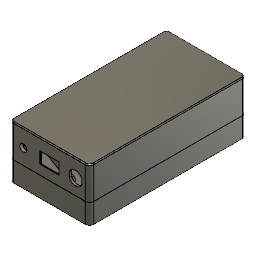
beltpack_pi_2s (Autodesk Fusion 360 design; units mm, degrees)
Autodesk Fusion 360 part; units mm, degrees
note: some values were not read from the file. Set by a fixed rule: which face or edge a step refers to.
sketch "case_form" plane through (0, 0, 0) normal (0, 0, 1) x (1, 0, 0)
  line L0 (0, 0) -> (87, 0)
  line L1 (87, 0) -> (87, 35)
  line L2 (87, 35) -> (0, 35)
  line L3 (0, 35) -> (0, 0)
  dimension "d5" = 87
  dimension "d6" = 35
  measures "d5" distance of L0.start
  measures "d6" distance of L0.start
extrude "Extrude1" add sketch "case_form" along normal blind 175 makes body 1
fillet "Fillet5" radius 2.5 4 edges at (87, 17.5, 175) (0, 17.5, 175) (87, 17.5, 0) (0, 17.5, 0) on bodies 1
shell "Shell1" thickness 2.4 outward yes removed faces 0 bodies 1
fillet "Fillet1" radius 1 8 edges at (-2.4, 37.4, 87.5) (-0.9648, 37.4, -0.9648) (43.5, 37.4, -2.4) (87.9648, 37.4, -0.9648) (89.4, 37.4, 87.5) (87.9648, 37.4, 175.9648) (43.5, 37.4, 177.4) (-0.9648, 37.4, 175.9648) on bodies 1
ref_plane "WorkPlane1" through (43.5, 0, 87.5) normal (0, -1, 0) x (1, 0, 0)
split "Split1" by plane through (43.5, 0, 87.5) normal (0, -1, 0) bodies 1 makes body 2 at (28.2, -2.4, 59.1667)
sketch "electronics" plane through (0, 35, 0) normal (0, -1, 0) x (1, 0, 0)
  line L0 (23, 152) -> (79, 152) construction
  line L1 (79, 152) -> (79, 67) construction
  line L2 (79, 67) -> (23, 67) construction
  line L3 (23, 67) -> (23, 152) construction
  circle A0 centre (26.5, 148.5) radius 3
  circle A1 centre (26.5, 148.5) radius 1
  circle A2 centre (75.5, 148.5) radius 3
  circle A3 centre (75.5, 148.5) radius 1
  circle A4 centre (26.5, 90.5) radius 3
  circle A5 centre (75.5, 90.5) radius 3
  circle A6 centre (75.5, 90.5) radius 1
  circle A7 centre (26.5, 90.5) radius 1
  line L4 (23, 40) -> (50, 40) construction
  line L5 (50, 40) -> (50, 24) construction
  line L6 (50, 24) -> (23, 24) construction
  line L7 (23, 24) -> (23, 40) construction
  circle A8 centre (25, 26) radius 3
  circle A9 centre (25, 26) radius 1
  circle A10 centre (48, 26) radius 3
  circle A11 centre (48, 26) radius 1
  arc A12 (0, 2.5) -> (2.5, 0) centre (2.5, 2.5) ccw
  line L8 (2.5, 0) -> (84.5, 0)
  arc A13 (84.5, 0) -> (87, 2.5) centre (84.5, 2.5) ccw
  line L9 (87, 2.5) -> (87, 172.5)
  arc A14 (87, 172.5) -> (84.5, 175) centre (84.5, 172.5) ccw
  line L10 (84.5, 175) -> (2.5, 175)
  arc A15 (2.5, 175) -> (0, 172.5) centre (2.5, 172.5) ccw
  line L11 (0, 172.5) -> (0, 2.5)
  arc A16 (1.5, 2.5) -> (2.5, 1.5) centre (2.5, 2.5) ccw
  line L12 (2.5, 1.5) -> (84.5, 1.5)
  arc A17 (84.5, 1.5) -> (85.5, 2.5) centre (84.5, 2.5) ccw
  line L13 (85.5, 2.5) -> (85.5, 172.5)
  arc A18 (85.5, 172.5) -> (84.5, 173.5) centre (84.5, 172.5) ccw
  line L14 (84.5, 173.5) -> (2.5, 173.5)
  arc A19 (2.5, 173.5) -> (1.5, 172.5) centre (2.5, 172.5) ccw
  line L15 (1.5, 172.5) -> (1.5, 2.5)
  line L16 (0, 172.5) -> (1.5, 172.5)
  line L17 (1.5, 172.5) -> (1.5, 170.5)
  line L18 (1.5, 170.5) -> (0, 170.5)
  line L19 (0, 170.5) -> (0, 172.5)
  line L20 (2.5, 175) -> (4.5, 175)
  line L21 (4.5, 175) -> (4.5, 173.5)
  line L22 (4.5, 173.5) -> (2.5, 173.5)
  line L23 (2.5, 173.5) -> (2.5, 175)
  arc A20 (0.4999, 2.5) -> (2.5, 0.4999) centre (2.5, 2.5) ccw
  line L24 (2.5, 0.4999) -> (84.5, 0.4999)
  arc A21 (84.5, 0.4999) -> (86.5001, 2.5) centre (84.5, 2.5) ccw
  line L25 (86.5001, 2.5) -> (86.5001, 172.5)
  arc A22 (86.5001, 172.5) -> (84.5, 174.5001) centre (84.5, 172.5) ccw
  line L26 (84.5, 174.5001) -> (2.5, 174.5001)
  arc A23 (2.5, 174.5001) -> (0.4999, 172.5) centre (2.5, 172.5) ccw
  line L27 (0.4999, 172.5) -> (0.4999, 2.5)
  line L28 (84.5, 175) -> (82.5, 175)
  line L29 (82.5, 175) -> (82.5, 138.5)
  line L30 (82.5, 138.5) -> (84.5, 138.5)
  line L31 (84.5, 138.5) -> (84.5, 175)
  line L32 (87, 172.5) -> (85.5, 172.5)
  line L33 (85.5, 172.5) -> (85.5, 170.5)
  line L34 (85.5, 170.5) -> (87, 170.5)
  line L35 (87, 170.5) -> (87, 172.5)
  line L36 (84.5, 0) -> (82.5, 0)
  line L37 (82.5, 0) -> (82.5, 1.5)
  line L38 (82.5, 1.5) -> (84.5, 1.5)
  line L39 (84.5, 1.5) -> (84.5, 0)
  line L40 (87, 2.5) -> (85.5, 2.5)
  line L41 (85.5, 2.5) -> (85.5, 4.5)
  line L42 (85.5, 4.5) -> (87, 4.5)
  line L43 (87, 4.5) -> (87, 2.5)
  line L44 (2.5, 0) -> (4.5, 0)
  line L45 (4.5, 0) -> (4.5, 1.5)
  line L46 (4.5, 1.5) -> (2.5, 1.5)
  line L47 (2.5, 1.5) -> (2.5, 0)
  line L48 (0, 2.5) -> (1.5, 2.5)
  line L49 (1.5, 2.5) -> (1.5, 4.5)
  line L50 (1.5, 4.5) -> (0, 4.5)
  line L51 (0, 4.5) -> (0, 2.5)
  line L52 (85.5, 135) -> (87, 135)
  line L53 (87, 135) -> (87, 130)
  line L54 (87, 130) -> (85.5, 130)
  line L55 (85.5, 130) -> (85.5, 135)
  line L56 (85.5, 45) -> (87, 45)
  line L57 (87, 45) -> (87, 40)
  line L58 (87, 40) -> (85.5, 40)
  line L59 (85.5, 40) -> (85.5, 45)
  line L60 (0, 135) -> (1.5, 135)
  line L61 (1.5, 135) -> (1.5, 130)
  line L62 (1.5, 130) -> (0, 130)
  line L63 (0, 130) -> (0, 135)
  line L64 (1.5, 45) -> (0, 45)
  line L65 (0, 45) -> (0, 40)
  line L66 (0, 40) -> (1.5, 40)
  line L67 (1.5, 40) -> (1.5, 45)
  line L68 (23, 63) -> (54, 63) construction
  line L69 (54, 63) -> (54, 44) construction
  line L70 (54, 44) -> (23, 44) construction
  line L71 (23, 44) -> (23, 63) construction
  circle A24 centre (26, 61) radius 1
  circle A25 centre (26, 61) radius 3
  circle A26 centre (51, 46) radius 1
  circle A27 centre (51, 46) radius 3
  dimension "d12" = 85
  dimension "d13" = 56
  dimension "d15" = 6
  dimension "d16" = 3.5
  dimension "d17" = 3.5
  dimension "d18" = 2
  dimension "d19" = 6
  dimension "d20" = 3.5
  dimension "d21" = 3.5
  dimension "d22" = 2
  dimension "d23" = 6
  dimension "d24" = 6
  dimension "d26" = 3.5
  dimension "d28" = 3.5
  dimension "d29" = 2
  dimension "d30" = 2
  dimension "d114" = 27
  dimension "d115" = 16
  dimension "d118" = 6
  dimension "d120" = 2
  dimension "d121" = 2
  dimension "d122" = 6
  dimension "d125" = 2
  dimension "d357" = 1.5
  dimension "d358" = 2
  dimension "d359" = 1.5
  dimension "d360" = 1.5
  dimension "d361" = 2
  dimension "d366" = 0.4999
  dimension "d375" = 2
  dimension "d376" = 2
  dimension "d377" = 2
  dimension "d378" = 1.5
  dimension "d379" = 1.5
  dimension "d380" = 2
  dimension "d381" = 2
  dimension "d382" = 1.5
  dimension "d383" = 1.5
  dimension "d384" = 2
  dimension "d419" = 5
  dimension "d420" = 40
  dimension "d422" = 5
  dimension "d423" = 85
  dimension "d425" = 1.5
  dimension "d426" = 5
  dimension "d427" = 40
  dimension "d428" = 5
  dimension "d429" = 1.5
  dimension "d430" = 85
  dimension "d490" = 58
  dimension "d491" = 58
  dimension "d492" = 26.5
  dimension "d493" = 26.5
  dimension "d494" = 22
  dimension "d495" = 19
  dimension "d496" = 31
  dimension "d497" = 2
  dimension "d498" = 6
  dimension "d499" = 2
  dimension "d500" = 2
  dimension "d501" = 6
  dimension "d502" = 2
  dimension "d503" = 3
  dimension "d504" = 3
  dimension "d505" = 4
  dimension "d507" = 2
  dimension "d508" = 4
  dimension "d509" = 2
  dimension "d510" = 2
  measures "d15" diameter of A0
  measures "d18" diameter of A1
  measures "d19" diameter of A2
  measures "d22" diameter of A3
  measures "d23" diameter of A4
  measures "d24" diameter of A5
  measures "d29" diameter of A6
  measures "d30" diameter of A7
  measures "d118" diameter of A8
  measures "d121" diameter of A9
  measures "d122" diameter of A10
  measures "d125" diameter of A11
  measures "d359" distance of origin
  measures "d378" distance of origin
  measures "d425" distance of origin
  measures "d427" distance of L10
  measures "d492" distance of origin L10
  measures "d493" distance of origin L11
  measures "d497" diameter of A24
  measures "d498" diameter of A25
  measures "d500" diameter of A26
  measures "d501" diameter of A27
  measures "d505" distance of L2 L68
  measures "d508" distance of L4 L70
sketch "oled_panel" plane through (0, 0, 177.4) normal (0, 0, 1) x (1, 0, 0)
  line L0 (2.5, 0) -> (84.5, 0)
  line L1 (29.5, 33.7) -> (57.5, 33.7)
  line L2 (57.5, 33.7) -> (57.5, 5.2)
  line L3 (57.5, 5.2) -> (29.5, 5.2)
  line L4 (29.5, 5.2) -> (29.5, 33.7)
  line L5 (32.5, 24) -> (54.5, 24)
  line L6 (54.5, 24) -> (54.5, 11)
  line L7 (54.5, 11) -> (32.5, 11)
  line L8 (32.5, 11) -> (32.5, 24)
  line L9 (43.5, 24) -> (43.5, 11) construction
  line L10 (54.5, 17.5) -> (32.5, 17.5) construction
  circle A0 centre (13.6, 17.5) radius 4
  circle A1 centre (73.4, 17.5) radius 7.75
  line L11 (28.5, 34.7) -> (20.7, 34.7)
  line L12 (20.7, 34.7) -> (20.7, 26.9)
  line L13 (20.7, 26.9) -> (28.5, 26.9)
  line L14 (28.5, 26.9) -> (28.5, 34.7)
  line L15 (24.6, 34.7) -> (24.6, 19.5918)
  line L16 (24.6, 19.5918) -> (24.6, 26.9) construction
  line L17 (20.7, 30.8) -> (28.5, 30.8) construction
  line L18 (58.5, 12) -> (66.3, 12)
  line L19 (66.3, 12) -> (66.3, 4.2)
  line L20 (66.3, 4.2) -> (58.5, 4.2)
  line L21 (58.5, 4.2) -> (58.5, 12)
  line L22 (62.4, 12) -> (62.4, 4.2) construction
  line L23 (66.3, 8.1) -> (58.5, 8.1) construction
  circle A2 centre (24.6, 30.8) radius 1.6
  circle A3 centre (24.6, 30.8) radius 1
  circle A4 centre (62.4, 8.1) radius 1.6
  circle A5 centre (62.4, 8.1) radius 1
  line L24 (66.25, 23.5) -> (80.55, 23.5)
  line L25 (80.55, 23.5) -> (80.55, 11.5)
  line L26 (80.55, 11.5) -> (66.25, 11.5)
  line L27 (66.25, 11.5) -> (66.25, 23.5)
  line L28 (66.25, 17.5) -> (80.55, 17.5) construction
  line L29 (73.4, 23.5) -> (73.4, 11.5) construction
  line L30 (7.3498, 14.0837) -> (9.2554, 11.7666)
  line L31 (9.2554, 11.7666) -> (7.7223, 10.4776)
  line L32 (7.7223, 10.4776) -> (5.8047, 12.8137)
  line L33 (5.8047, 12.8137) -> (7.3498, 14.0837)
  circle A6 centre (13.6, 17.5) radius 8.2 construction
  line L34 (8.3026, 12.9251) -> (6.7635, 11.6457) construction
  line L35 (6.5772, 13.4487) -> (8.4888, 11.1221) construction
  line L36 (30, 8.45) -> (35.5, 8.45)
  line L37 (35.5, 8.45) -> (35.5, 5.7)
  line L38 (35.5, 5.7) -> (30, 5.7)
  line L39 (30, 5.7) -> (30, 8.45)
  line L40 (79, 35) -> (23, 35)
  line L41 (43.5, 0) -> (43.5, 35)
  line L42 (84.5, 0) -> (84.5, 36.4)
  line L43 (84.5, 36.4) -> (2.5, 36.4)
  line L44 (2.5, 36.4) -> (2.5, 0)
  line L45 (58.5, 34.7) -> (58.5, 4.2)
  line L46 (58.5, 4.2) -> (28.5, 4.2)
  line L47 (28.5, 4.2) -> (28.5, 34.7)
  line L48 (28.5, 34.7) -> (58.5, 34.7)
  line L49 (51.5, 8.45) -> (57, 8.45)
  line L50 (57, 8.45) -> (57, 5.7)
  line L51 (57, 5.7) -> (51.5, 5.7)
  line L52 (51.5, 5.7) -> (51.5, 8.45)
  line L53 (38.15, 7.7) -> (48.85, 7.7)
  line L54 (48.85, 7.7) -> (48.85, 5.7)
  line L55 (48.85, 5.7) -> (38.15, 5.7)
  line L56 (38.15, 5.7) -> (38.15, 7.7)
  line L57 (30, 33.2) -> (35.5, 33.2)
  line L58 (35.5, 33.2) -> (35.5, 30.45)
  line L59 (35.5, 30.45) -> (30, 30.45)
  line L60 (30, 30.45) -> (30, 33.2)
  line L61 (51.5, 33.2) -> (57, 33.2)
  line L62 (57, 33.2) -> (57, 30.45)
  line L63 (57, 30.45) -> (51.5, 30.45)
  line L64 (51.5, 30.45) -> (51.5, 33.2)
  line L65 (19.2644, 29.4032) -> (25.9968, 25.4644)
  line L66 (25.9968, 25.4644) -> (29.9356, 32.1968)
  line L67 (29.9356, 32.1968) -> (23.2032, 36.1356)
  line L68 (23.2032, 36.1356) -> (19.2644, 29.4032)
  line L69 (27.9662, 28.8306) -> (21.2338, 32.7694) construction
  line L70 (22.6306, 27.4338) -> (26.5694, 34.1662) construction
  circle A7 centre (24.6, 30.8) radius 1.6
  line L71 (57.0638, 6.736) -> (63.7686, 2.7504)
  line L72 (63.7686, 2.7504) -> (67.7338, 9.4635)
  line L73 (67.7338, 9.4635) -> (61.0338, 13.4501)
  line L74 (61.0338, 13.4501) -> (57.0638, 6.736)
  line L75 (59.0488, 10.0931) -> (65.7512, 6.1069) construction
  line L76 (60.4162, 4.7432) -> (64.3838, 11.4568) construction
  circle A8 centre (62.4, 8.1) radius 1.6
  line L77 (25.9968, 25.4644) -> (57.0918, 6.7188)
  line L78 (57.0918, 6.7188) -> (61.0338, 13.4501)
  line L79 (61.0338, 13.4501) -> (29.936, 32.1974)
  line L80 (29.936, 32.1974) -> (25.9968, 25.4644)
  line L81 (73.4, 0) -> (73.4, 35) construction
  circle A9 centre (73.4, 17.5) radius 10.5 construction
  line L82 (62.4, 12) -> (66.3, 8.1)
  circle A10 centre (13.6, 17.5) radius 10
  dimension "d31" = 28
  dimension "d32" = 28.5
  dimension "d33" = 22
  dimension "d34" = 13
  dimension "d36" = 8
  dimension "d38" = 1
  dimension "d39" = 15.5
  dimension "d40" = 7.8
  dimension "d41" = 7.8
  dimension "d42" = 7.8
  dimension "d43" = 7.8
  dimension "d44" = 3.2
  dimension "d45" = 2
  dimension "d46" = 3.2
  dimension "d47" = 2
  dimension "d50" = 5.8
  dimension "d51" = 14.3
  dimension "d52" = 12
  dimension "d53" = 3
  dimension "d54" = 2
  dimension "d55" = 16.4
  dimension "d57" = 5.5
  dimension "d58" = 2.75
  dimension "d59" = 0.5
  dimension "d60" = 0.5
  dimension "d80" = 8
  dimension "d451" = 5.5
  dimension "d452" = 2.75
  dimension "d453" = 0.5
  dimension "d454" = 0.5
  dimension "d455" = 10.7
  dimension "d456" = 2
  dimension "d457" = 0.5
  dimension "d458" = 5.5
  dimension "d459" = 2.75
  dimension "d460" = 0.5
  dimension "d461" = 0.5
  dimension "d462" = 5.5
  dimension "d463" = 2.75
  dimension "d464" = 0.5
  dimension "d465" = 0.5
  dimension "d472" = 7.8
  dimension "d473" = 7.8
  dimension "d474" = 3.2
  dimension "d475" = 7.8
  dimension "d476" = 7.8
  dimension "d477" = 3.2
  dimension "d479" = 7.8
  dimension "d487" = 11.1
  dimension "d488" = 21
  dimension "d512" = 20
  measures "d32" distance of origin
  measures "d34" distance of origin
  measures "d36" diameter of A0
  measures "d38" distance of L2
  measures "d39" diameter of A1
  measures "d44" diameter of A2
  measures "d45" diameter of A3
  measures "d46" diameter of A4
  measures "d47" diameter of A5
  measures "d50" distance of L3 L7
  measures "d52" distance of origin
  measures "d55" diameter of A6
  measures "d59" distance of L3 L38
  measures "d60" distance of L4 L39
  measures "d453" distance of L3 L51
  measures "d454" distance of L2 L50
  measures "d457" distance of L3 L55
  measures "d460" distance of L1 L57
  measures "d461" distance of L4 L60
  measures "d464" distance of L1 L61
  measures "d465" distance of L2 L62
  measures "d472" distance of origin
  measures "d473" distance of origin
  measures "d474" diameter of A7
  measures "d477" diameter of A8
  measures "d479" distance of L77 L79
  measures "d488" diameter of A9
  measures "d512" diameter of A10
extrude "Extrude2" cut sketch "oled_panel" against normal up to surface (2.4 mm away) contours L5 L8 L41 L77 | L5 L6 L7 L41 L77 L79 | L5 L6 L79 | L7 L41 L77 | L7 L8 L41 L77 | A1 L24 L25 L26 L27 | A1 L26 | A1 L24 | A0 bodies 1
extrude "Extrude3" cut sketch "electronics" against normal blind 1 contours A1 | A3 | A6 | A7 | A9 | A11 | A24 | A26 bodies 1
extrude "Extrude4" add sketch "electronics" along normal blind 5 contours A0 | A2 | A4 | A5 | A8 | A10 | A25 | A27 bodies 1
extrude "Extrude7" cut sketch "oled_panel" along normal blind 1.4 from surface at -2.4 contours L1 L4 L41 L57 L58 L59 L60 L67 L79 | L1 L2 L5 L6 L41 L79 | L4 L66 L67 L80 | L5 L41 L79 | L4 L5 L8 L41 L59 L60 L66 L77 L79 L80 | L2 L6 L7 L49 L50 L74 L77 L79 | L57 L58 L59 L60 L79 | L59 L60 L79 | L3 L4 L7 L8 L41 L53 L55 L56 L77 | L2 L71 L74 L77 L78 | L2 L71 L78 | L2 L3 L7 L41 L49 L50 L51 L52 L53 L54 L55 L71 L77 | L49 L50 L77 | L49 L50 L51 L52 L77 | L41 L53 L54 L55 | L41 L53 L55 L56 | L36 L37 L38 L39 | L61 L62 L63 L64 bodies 1
extrude "Extrude8" add sketch "oled_panel" against normal blind 2.6 from surface at -2.4 contours L1 L4 L14 L41 L47 L48 L67 | L1 L2 L41 L45 L48 L79 | L4 L14 L47 L66 L67 L80 | L4 L14 L47 L66 L77 L80 | L11 L14 L47 L67 | L11 L13 L14 L15 A2 L47 L66 L67 A7 L80 | L2 L21 L45 L74 L79 | L3 L4 L41 L46 L47 L77 | L13 L14 L47 L66 L80 | L2 L21 L45 L74 L78 | L11 L12 L13 L15 A2 L65 L68 A7 | L2 L21 L45 L71 L78 | L18 L21 L45 L74 L78 | L18 L21 L45 L74 | L2 L3 L21 L41 L45 L46 L71 | L11 L12 L68 | L15 A2 A3 A7 | L15 A2 A3 A7 | L18 L19 L20 L21 L45 L71 L72 L78 L82 | L12 L13 L65 | L20 L21 L45 L71 | L19 L20 L72 | A4 A8 bodies 1
fillet "Fillet3" radius 2 9 edges at (28.5, 4.2, 173.7) (66.3, 4.2, 173.7) (20.7, 26.9, 173.7) (58.5, 12, 173.7) (58.5, 34.7, 173.7) (28.5, 26.9, 173.7) (20.7, 34.7, 173.7) (62.4, 12, 173.7) (66.3, 8.1, 173.7) on bodies 1
extrude "Extrude36" add sketch "oled_panel" against normal blind 2.5 contours L57 L58 L59 L60 L79 | L59 L60 L79 | L49 L50 L77 | L49 L50 L51 L52 L77 | L36 L37 L38 L39 | L61 L62 L63 L64 bodies 1
fillet "Fillet18" radius 1 16 edges at (51.5, 8.45, 175.65) (57, 8.45, 175.65) (51.5, 5.7, 175.65) (57, 5.7, 175.65) (35.5, 8.45, 175.65) (35.5, 5.7, 175.65) (30, 8.45, 175.65) (30, 5.7, 175.65) (30, 30.45, 175.65) (35.5, 30.45, 175.65) (35.5, 33.2, 175.65) (30, 33.2, 175.65) (51.5, 33.2, 175.65) (51.5, 30.45, 175.65) (57, 33.2, 175.65) (57, 30.45, 175.65) on bodies 1
sketch "headset_panel" plane through (0, 0, -2.4) normal (0, 0, -1) x (-1, 0, 0)
  line L0 (-84.5, 0) -> (-2.5, 0)
  line L1 (-39, 31.7) -> (-8, 31.7) construction
  line L2 (-8, 31.7) -> (-8, 5.7) construction
  line L3 (-8, 5.7) -> (-39, 5.7) construction
  line L4 (-39, 5.7) -> (-39, 31.7) construction
  line L5 (-87, 0) -> (-87, 35)
  line L6 (-39, 18.7) -> (-8, 18.7) construction
  line L7 (-23.5, 31.7) -> (-23.5, 5.7) construction
  circle A0 centre (-23.5, 18.7) radius 12.3
  circle A1 centre (-35.6, 8.9) radius 1.6
  circle A2 centre (-11.4, 28.5) radius 1.6
  circle A3 centre (-47, 18.7) radius 4.1
  line L8 (0, 0) -> (0, 35)
  line L9 (-2.5, 0) -> (-2.5, 36.4)
  line L10 (-2.5, 36.4) -> (-84.5, 36.4)
  line L11 (-84.5, 36.4) -> (-84.5, 0)
  line L12 (-30, 0) -> (-24, 0)
  line L13 (-24, 0) -> (-24, 5.2)
  line L14 (-24, 5.2) -> (-30, 5.2)
  line L15 (-30, 5.2) -> (-30, 0)
  line L16 (-8, -2) -> (-79, -2)
  line L17 (-79, -2) -> (-79, 0)
  line L18 (-79, 0) -> (-8, 0)
  line L19 (-8, 0) -> (-8, -2)
  line L20 (-24, 0) -> (-30, 0)
  line L21 (-30, 0) -> (-30, -2)
  line L22 (-30, -2) -> (-24, -2)
  line L23 (-24, -2) -> (-24, 0)
  line L24 (-79, -2) -> (-8, -2)
  line L25 (-8, -2) -> (-8, -7)
  line L26 (-8, -7) -> (-79, -7)
  line L27 (-79, -7) -> (-79, -2)
  line L28 (-10, -7) -> (-77, -7)
  line L29 (-77, -7) -> (-77, -1)
  line L30 (-77, -1) -> (-10, -1)
  line L31 (-10, -1) -> (-10, -7)
  dimension "d82" = 31
  dimension "d83" = 26
  dimension "d89" = 24.6
  dimension "d90" = 3.2
  dimension "d91" = 3.2
  dimension "d92" = 3.4
  dimension "d93" = 3.2
  dimension "d94" = 3.2
  dimension "d95" = 3.4
  dimension "d96" = 8.2
  dimension "d101" = 8
  dimension "d102" = 8
  dimension "d230" = 6
  dimension "d231" = 5.2
  dimension "d302" = 4.7
  dimension "d308" = 24
  dimension "d350" = 71
  dimension "d351" = 2
  dimension "d398" = 5
  dimension "d399" = 67
  dimension "d401" = 6
  dimension "d450" = 6
  measures "d82" distance of L8.start
  measures "d83" distance of L8.start
  measures "d89" diameter of A0
  measures "d90" diameter of A1
  measures "d91" distance of L3
  measures "d92" distance of L4
  measures "d93" diameter of A2
  measures "d94" distance of L1
  measures "d95" distance of L2
  measures "d96" diameter of A3
  measures "d230" distance of L8.start
  measures "d231" distance of L8.start
  measures "d302" distance of L8.start L10
  measures "d308" distance of L8 L13
  measures "d399" distance of L29 L31
  measures "d401" distance of L28 L30
  measures "d450" distance of L21 L23
extrude "Extrude9" cut sketch "headset_panel" against normal up to surface (2.4 mm away) contours L0 L12 L13 L14 L15 L18 L20 | A0 | A1 | A2 | A3 bodies 1
sketch "mounting bosses" plane through (0, -2.4, 0) normal (0, -1, 0) x (1, 0, 0)
  arc A0 (-2.4, 2.5) -> (2.5, -2.4) centre (2.5, 2.5) ccw
  line L0 (2.5, -2.4) -> (84.5, -2.4)
  arc A1 (84.5, -2.4) -> (89.4, 2.5) centre (84.5, 2.5) ccw
  line L1 (89.4, 2.5) -> (89.4, 172.5)
  arc A2 (89.4, 172.5) -> (84.5, 177.4) centre (84.5, 172.5) ccw
  line L2 (84.5, 177.4) -> (2.5, 177.4)
  arc A3 (2.5, 177.4) -> (-2.4, 172.5) centre (2.5, 172.5) ccw
  line L3 (-2.4, 172.5) -> (-2.4, 2.5)
  line L4 (0, 2.5) -> (0, 172.5)
  line L5 (84.5, 0) -> (2.5, 0)
  line L6 (17.6, 175) -> (9.6, 175)
  line L7 (2.5, 175) -> (84.5, 175)
  circle A4 centre (2.6, 160) radius 2.3
  line L8 (0, 165) -> (7.6, 165)
  line L9 (7.6, 165) -> (7.6, 155)
  line L10 (7.6, 155) -> (0, 155)
  line L11 (0, 155) -> (0, 165)
  line L12 (3.8, 155) -> (3.8, 165) construction
  line L13 (0, 20) -> (7.6, 20)
  line L14 (7.6, 20) -> (7.6, 10)
  line L15 (7.6, 10) -> (0, 10)
  line L16 (0, 10) -> (0, 20)
  circle A5 centre (2.6, 15) radius 2.3
  line L17 (3.8, 10) -> (3.8, 20) construction
  circle A6 centre (2.6, 87.5) radius 2.3
  line L18 (0, 92.5) -> (7.6, 92.5)
  line L19 (7.6, 92.5) -> (7.6, 82.5)
  line L20 (7.6, 82.5) -> (0, 82.5)
  line L21 (0, 82.5) -> (0, 92.5)
  line L22 (3.8, 82.5) -> (3.8, 92.5) construction
  circle A7 centre (84.4, 15) radius 2.3
  line L23 (87, 10) -> (79.4, 10)
  line L24 (79.4, 10) -> (79.4, 20)
  line L25 (79.4, 20) -> (87, 20)
  line L26 (87, 20) -> (87, 10)
  line L27 (87, 2.5) -> (87, 172.5)
  line L28 (83.2, 10) -> (83.2, 20) construction
  circle A8 centre (84.4, 87.5) radius 2.3
  line L29 (87, 82.5) -> (79.4, 82.5)
  line L30 (79.4, 82.5) -> (79.4, 92.5)
  line L31 (79.4, 92.5) -> (87, 92.5)
  line L32 (87, 92.5) -> (87, 82.5)
  line L33 (83.2, 82.5) -> (83.2, 92.5) construction
  line L34 (87, 165) -> (79.4, 165)
  line L35 (79.4, 165) -> (79.4, 155)
  line L36 (79.4, 155) -> (87, 155)
  line L37 (87, 155) -> (87, 165)
  circle A9 centre (84.4, 160) radius 2.3
  line L38 (83.2, 155) -> (83.2, 165) construction
  line L39 (30, 0) -> (84.5, 0)
  line L40 (2.5, 0) -> (24, 0)
  line L41 (2.5, 0.6) -> (84.5, 0.6)
  arc A10 (84.5, 0.6) -> (86.4, 2.5) centre (84.5, 2.5) ccw
  line L42 (86.4, 2.5) -> (86.4, 172.5)
  arc A11 (86.4, 172.5) -> (84.5, 174.4) centre (84.5, 172.5) ccw
  line L43 (84.5, 174.4) -> (2.5, 174.4)
  arc A12 (2.5, 174.4) -> (0.6, 172.5) centre (2.5, 172.5) ccw
  line L44 (0.6, 172.5) -> (0.6, 2.5)
  arc A13 (0.6, 2.5) -> (2.5, 0.6) centre (2.5, 2.5) ccw
  dimension "d149" = 4.6
  dimension "d150" = 5
  dimension "d151" = 7.6
  dimension "d152" = 10
  dimension "d153" = 10
  dimension "d160" = 7.6
  dimension "d161" = 10
  dimension "d162" = 4.6
  dimension "d163" = 5
  dimension "d164" = 10
  dimension "d166" = 4.6
  dimension "d167" = 5
  dimension "d168" = 10
  dimension "d169" = 7.6
  dimension "d173" = 4.6
  dimension "d174" = 5
  dimension "d175" = 7.6
  dimension "d176" = 10
  dimension "d178" = 4.6
  dimension "d179" = 5
  dimension "d180" = 10
  dimension "d181" = 7.6
  dimension "d182" = 7.6
  dimension "d183" = 10
  dimension "d184" = 4.6
  dimension "d185" = 5
  dimension "d186" = 10
  dimension "d188" = 3
  measures "d149" diameter of A4
  measures "d150" distance of L3
  measures "d153" distance of L7 L8
  measures "d162" diameter of A5
  measures "d163" distance of L3
  measures "d164" distance of L5
  measures "d166" diameter of A6
  measures "d173" diameter of A7
  measures "d174" distance of L1
  measures "d176" distance of origin
  measures "d178" diameter of A8
  measures "d180" distance of origin
  measures "d181" distance of origin
  measures "d182" distance of origin
  measures "d183" distance of origin
  measures "d184" diameter of A9
  measures "d185" distance of L1 origin
  measures "d186" distance of L7
  measures "d188" distance of L0
extrude "Extrude12" add sketch "mounting bosses" against normal blind 1.6 separate body contours L13 L14 L15 A5 L44 | L8 L9 L10 L13 L14 L15 L18 L19 L20 L23 L24 L25 L29 L30 L31 L34 L35 L36 L41 A10 L42 A11 L43 A12 L44 A13 | A5 L44 | A6 L18 L19 L20 L44 | A6 L44 | A4 L8 L9 L10 L44 | A4 L44 | A7 L23 L24 L25 L42 | A7 L42 | A8 L29 L30 L31 L42 | L34 L35 L36 A9 L42 | A8 L42 | A9 L42 picked at (2.2057, 15.7049) picked at (3.6343, 87.5501) picked at (2.0333, 160) picked at (85.7042, 15.7265) picked at (85.3112, 88.0822) picked at (84.8425, 160) makes body 3
extrude "Extrude11" add sketch "mounting bosses" against normal blind 15 from surface at -4.5 contours L4 L13 L15 L16 A5 L44 | L13 L14 L15 A5 L44 | L4 A6 L18 L20 L21 L44 | A6 L18 L19 L20 L44 | L4 A4 L8 L10 L11 L44 | A4 L8 L9 L10 L44 | A7 L23 L25 L26 L27 L42 | A7 L23 L24 L25 L42 | L27 A8 L29 L31 L32 L42 | A8 L29 L30 L31 L42 | L34 L35 L36 A9 L42 | L27 L34 L36 L37 A9 L42 bodies 1
chamfer "Chamfer2" distance 7.5 angle 45 6 edges at (7.6, 17.1, 160) (7.6, 17.1, 15) (7.6, 17.1, 87.5) (79.4, 17.1, 160) (79.4, 17.1, 87.5) (79.4, 17.1, 15) measured on face at (6.7, 17.1, 160) measured on face at (6.7, 17.1, 15) measured on face at (6.7, 17.1, 87.5) measured on face at (80.3, 17.1, 160) measured on face at (80.3, 17.1, 87.5) measured on face at (80.3, 17.1, 15) on bodies 1
fillet "Fillet6" radius 2 24 edges at (7.6, 5.85, 155) (7.6, 5.85, 165) (0, 9.6, 165) (0, 9.6, 155) (0, 9.6, 20) (7.6, 5.85, 20) (7.6, 5.85, 10) (0, 9.6, 10) (0, 9.6, 82.5) (7.6, 5.85, 82.5) (7.6, 5.85, 92.5) (0, 9.6, 92.5) (87, 9.6, 165) (79.4, 5.85, 165) (79.4, 5.85, 155) (87, 9.6, 92.5) (79.4, 5.85, 92.5) (79.4, 5.85, 82.5) (87, 9.6, 20) (79.4, 5.85, 20) (79.4, 5.85, 10) (87, 9.6, 155) (87, 9.6, 82.5) (87, 9.6, 10) on bodies 1
move_body "Move3" bodies 3 to x (1, 0, 0) y (0, 1, 0) z (0, 0, 1) at (0, 2.8, 0)
sketch "battery_bottom" plane through (0, 0.4, 0) normal (0, -1, 0) x (1, 0, 0)
  arc A0 (0.6, 2.5) -> (2.5, 0.6) centre (2.5, 2.5) ccw
  line L0 (2.5, 0.6) -> (84.5, 0.6)
  arc A1 (84.5, 0.6) -> (86.4, 2.5) centre (84.5, 2.5) ccw
  line L1 (86.4, 2.5) -> (86.4, 172.5)
  arc A2 (86.4, 172.5) -> (84.5, 174.4) centre (84.5, 172.5) ccw
  line L2 (84.5, 174.4) -> (2.5, 174.4)
  arc A3 (2.5, 174.4) -> (0.6, 172.5) centre (2.5, 172.5) ccw
  line L3 (0.6, 172.5) -> (0.6, 2.5)
  line L4 (0.6, 17.6) -> (5.4, 17.6)
  line L5 (5.4, 17.6) -> (5.4, 12.4)
  line L6 (5.4, 12.4) -> (0.6, 12.4)
  line L7 (0.6, 12.4) -> (0.6, 17.6)
  line L8 (3, 12.4) -> (3, 17.6) construction
  line L9 (0.6, 90.1) -> (5.4, 90.1)
  line L10 (5.4, 90.1) -> (5.4, 84.9)
  line L11 (5.4, 84.9) -> (0.6, 84.9)
  line L12 (0.6, 84.9) -> (0.6, 90.1)
  line L13 (3, 90.1) -> (3, 84.9) construction
  line L14 (0.6, 162.6) -> (5.4, 162.6)
  line L15 (5.4, 162.6) -> (5.4, 157.4)
  line L16 (5.4, 157.4) -> (0.6, 157.4)
  line L17 (0.6, 157.4) -> (0.6, 162.6)
  line L18 (3, 157.4) -> (3, 162.6) construction
  line L19 (86.4, 162.6) -> (81.6, 162.6)
  line L20 (81.6, 162.6) -> (81.6, 157.4)
  line L21 (81.6, 157.4) -> (86.4, 157.4)
  line L22 (86.4, 157.4) -> (86.4, 162.6)
  line L23 (84, 162.6) -> (84, 157.4) construction
  line L24 (86.4, 90.1) -> (81.6, 90.1)
  line L25 (81.6, 90.1) -> (81.6, 84.9)
  line L26 (81.6, 84.9) -> (86.4, 84.9)
  line L27 (86.4, 84.9) -> (86.4, 90.1)
  line L28 (84, 84.9) -> (84, 90.1) construction
  line L29 (86.4, 17.6) -> (81.6, 17.6)
  line L30 (81.6, 17.6) -> (81.6, 12.4)
  line L31 (81.6, 12.4) -> (86.4, 12.4)
  line L32 (86.4, 12.4) -> (86.4, 17.6)
  line L33 (84, 12.4) -> (84, 17.6) construction
  line L34 (86.6, 174.4) -> (0.6, 174.4)
  line L35 (0.6, 174.4) -> (0.6, 168.4)
  line L36 (0.6, 168.4) -> (86.6, 168.4)
  line L37 (86.6, 168.4) -> (86.6, 174.4)
  line L38 (30, 0.6) -> (24, 0.6)
  line L39 (24, 0.6) -> (24, 8.1)
  line L40 (24, 8.1) -> (30, 8.1)
  line L41 (30, 8.1) -> (30, 0.6)
  line L42 (0, 2.5) -> (0, 172.5)
  line L43 (0.6, 6) -> (6, 0.6)
  line L44 (81, 0.6) -> (86.4, 6)
  line L45 (0.6, 46.1) -> (2.6, 46.1)
  line L46 (2.6, 46.1) -> (2.6, 39.1)
  line L47 (2.6, 39.1) -> (0.6, 39.1)
  line L48 (0.6, 39.1) -> (0.6, 46.1)
  line L49 (0.6, 136.1) -> (2.6, 136.1)
  line L50 (2.6, 136.1) -> (2.6, 129.1)
  line L51 (2.6, 129.1) -> (0.6, 129.1)
  line L52 (0.6, 129.1) -> (0.6, 136.1)
  line L53 (86.4, 39.1) -> (84.4, 39.1)
  line L54 (84.4, 39.1) -> (84.4, 46.1)
  line L55 (84.4, 46.1) -> (86.4, 46.1)
  line L56 (86.4, 46.1) -> (86.4, 39.1)
  line L57 (86.4, 136.1) -> (84.4, 136.1)
  line L58 (84.4, 136.1) -> (84.4, 129.1)
  line L59 (84.4, 129.1) -> (86.4, 129.1)
  line L60 (86.4, 129.1) -> (86.4, 136.1)
  dimension "d194" = 5.2
  dimension "d195" = 4.8
  dimension "d199" = 5.2
  dimension "d200" = 4.8
  dimension "d201" = 5.2
  dimension "d202" = 4.8
  dimension "d203" = 5.2
  dimension "d204" = 4.8
  dimension "d205" = 4.8
  dimension "d206" = 5.2
  dimension "d207" = 5.2
  dimension "d208" = 4.8
  dimension "d210" = 6
  dimension "d211" = 86
  dimension "d303" = 6
  dimension "d304" = 7.5
  dimension "d309" = 24
  dimension "d391" = 5.4
  dimension "d392" = 5.4
  dimension "d393" = 5.4
  dimension "d394" = 5.4
  dimension "d432" = 7
  dimension "d433" = 2
  dimension "d435" = 38.5
  dimension "d436" = 7
  dimension "d437" = 2
  dimension "d438" = 83
  dimension "d440" = 7
  dimension "d441" = 2
  dimension "d442" = 7
  dimension "d443" = 2
  dimension "d444" = 38.5
  dimension "d445" = 83
  measures "d200" distance of origin
  measures "d202" distance of origin
  measures "d290" distance of origin
  measures "d303" distance of origin
  measures "d304" distance of origin
  measures "d309" distance of L39 L42
  measures "d391" distance of L3
  measures "d392" distance of L0
  measures "d393" distance of L0
  measures "d394" distance of L1 origin
  measures "d433" distance of origin
  measures "d435" distance of L0
  measures "d437" distance of origin
  measures "d444" distance of origin
extrude "Extrude14" cut sketch "battery_bottom" against normal up to surface (1.6 mm away) contours L3 L4 L5 L6 L7 | L3 L9 L10 L11 L12 | L1 L29 L30 L31 L32 | L3 L14 L15 L16 L17 | L1 L24 L25 L26 L27 | L1 L19 L20 L21 L22 bodies 3
extrude "Extrude15" cut sketch "battery_bottom" against normal up to surface (1.6 mm away) contours L1 A2 L2 A3 L3 L34 L35 L36 bodies 3
fillet "Fillet7" radius 2.5 26 edges at (0.6, 1.2, 17.6) (5.4, 1.2, 17.6) (5.4, 1.2, 12.4) (0.6, 1.2, 12.4) (5.4, 1.2, 84.9) (5.4, 1.2, 90.1) (0.6, 1.2, 90.1) (0.6, 1.2, 84.9) (0.6, 1.2, 162.6) (5.4, 1.2, 162.6) (5.4, 1.2, 157.4) (0.6, 1.2, 157.4) (86.4, 1.2, 162.6) (81.6, 1.2, 162.6) (81.6, 1.2, 157.4) (86.4, 1.2, 157.4) (86.4, 1.2, 84.9) (81.6, 1.2, 84.9) (81.6, 1.2, 90.1) (86.4, 1.2, 90.1) (86.4, 1.2, 12.4) (81.6, 1.2, 12.4) (81.6, 1.2, 17.6) (86.4, 1.2, 17.6) (86.4, 1.2, 168.4) (0.6, 1.2, 168.4) on bodies 3
extrude "Extrude16" add 1 faces at (28.2, -2.4, 59.1667) along direction (0, -1, 0) blind 20.6 on bodies 2 bodies 2
shell "Shell2" thickness 2.4 removed faces 1 at (58.8, 0, 115.8333) on bodies 2
sketch "battery_conn_hole" plane through (0, 0, -2.4) normal (0, 0, -1) x (-1, 0, 0)
  line L0 (-2.5, 0) -> (-84.5, 0)
  line L1 (-84.5, 0) -> (-84.5, -23)
  line L2 (-84.5, -23) -> (-2.5, -23)
  line L3 (-2.5, -23) -> (-2.5, 0)
  line L4 (-84.5, -14.5) -> (-2.5, -14.5679) construction
  line L5 (-79, 0) -> (-8, 0) construction
  line L6 (-8, 0) -> (-8, -14.1) construction
  line L7 (-8, -14.1) -> (-79, -14.1) construction
  line L8 (-79, -14.1) -> (-79, 0) construction
  line L9 (-72.5, -2) -> (-14.5, -2)
  line L10 (-14.5, -2) -> (-14.5, 0)
  line L11 (-14.5, 0) -> (-72.5, 0)
  line L12 (-72.5, 0) -> (-72.5, -2)
  line L13 (-10, -2) -> (-10, -12.1)
  line L14 (-10, -12.1) -> (-77, -12.1)
  line L15 (-77, -12.1) -> (-77, -2)
  line L16 (-77, -2) -> (-10, -2)
  line L17 (-77, -7.05) -> (-10, -7.05)
  line L18 (-10, -7.05) -> (-10, 0)
  line L19 (-10, 0) -> (-77, 0)
  line L20 (-77, 0) -> (-77, -7.05)
  line L21 (-79, 0) -> (-78.75, 0)
  line L22 (-78.75, 0) -> (-78.75, -7)
  line L23 (-78.75, -7) -> (-79, -7)
  line L24 (-79, -7) -> (-79, 0)
  line L25 (-79, -7) -> (-76.9, -7)
  line L26 (-76.9, -7) -> (-76.9, -6.75)
  line L27 (-76.9, -6.75) -> (-79, -6.75)
  line L28 (-79, -6.75) -> (-79, -7)
  line L29 (-8, 0) -> (-8.25, 0)
  line L30 (-8.25, 0) -> (-8.25, -7)
  line L31 (-8.25, -7) -> (-8, -7)
  line L32 (-8, -7) -> (-8, 0)
  line L33 (-8, -7) -> (-10.1, -7)
  line L34 (-10.1, -7) -> (-10.1, -6.75)
  line L35 (-10.1, -6.75) -> (-8, -6.75)
  line L36 (-8, -6.75) -> (-8, -7)
  dimension "d223" = 8.5
  dimension "d224" = 14.1
  dimension "d225" = 71
  dimension "d226" = 2
  dimension "d355" = 58
  dimension "d356" = 2
  dimension "d406" = 0.25
  dimension "d407" = 7
  dimension "d408" = 2.1
  dimension "d409" = 0.25
  dimension "d410" = 0.25
  dimension "d411" = 7
  dimension "d412" = 2.1
  dimension "d413" = 0.25
  dimension "d418" = 2
  measures "d223" distance of origin
  measures "d224" distance of origin
  measures "d226" distance of L6
  measures "d356" distance of origin
  measures "d407" distance of origin
extrude "Extrude17" cut sketch "battery_conn_hole" against normal up to surface (2.4 mm away) contours L0 L9 L10 L11 L12 L16 L19 | L9 L13 L15 L16 L17 L18 L20 L25 L26 L27 L33 L34 L35 | L13 L18 L33 L34 L35 | L13 L14 L15 L17 | L15 L20 L25 L26 L27 bodies 2
fillet "Fillet8" radius 5 4 edges at (10, -12.1, -1.2) (10, -2, -1.2) (77, -2, -1.2) (77, -12.1, -1.2) on bodies 2
sketch "battery_screw" plane through (0, -23, 0) normal (0, -1, 0) x (1, 0, 0)
  arc A0 (-2.4, 2.5) -> (2.5, -2.4) centre (2.5, 2.5) ccw
  line L0 (2.5, -2.4) -> (84.5, -2.4)
  arc A1 (84.5, -2.4) -> (89.4, 2.5) centre (84.5, 2.5) ccw
  line L1 (89.4, 2.5) -> (89.4, 172.5)
  arc A2 (89.4, 172.5) -> (84.5, 177.4) centre (84.5, 172.5) ccw
  line L2 (84.5, 177.4) -> (2.5, 177.4)
  arc A3 (2.5, 177.4) -> (-2.4, 172.5) centre (2.5, 172.5) ccw
  line L3 (-2.4, 172.5) -> (-2.4, 2.5)
  circle A4 centre (2.6, 15) radius 2.3
  line L4 (-0.9, 18.5) -> (6.1, 18.5)
  line L5 (6.1, 18.5) -> (6.1, 11.5)
  line L6 (6.1, 11.5) -> (-0.9, 11.5)
  line L7 (-0.9, 11.5) -> (-0.9, 18.5)
  line L8 (2.6, 18.5) -> (2.6, 11.5) construction
  line L9 (-0.9, 15) -> (6.1, 15) construction
  circle A5 centre (2.6, 87.5) radius 2.3
  line L10 (-0.9, 91) -> (6.1, 91)
  line L11 (6.1, 91) -> (6.1, 84)
  line L12 (6.1, 84) -> (-0.9, 84)
  line L13 (-0.9, 84) -> (-0.9, 91)
  line L14 (-0.9, 87.5) -> (6.1, 87.5) construction
  line L15 (2.6, 91) -> (2.6, 84) construction
  circle A6 centre (2.6, 160) radius 2.3
  line L16 (-0.9, 163.5) -> (6.1, 163.5)
  line L17 (6.1, 163.5) -> (6.1, 156.5)
  line L18 (6.1, 156.5) -> (-0.9, 156.5)
  line L19 (-0.9, 156.5) -> (-0.9, 163.5)
  line L20 (-0.9, 160) -> (6.1, 160) construction
  line L21 (2.6, 163.5) -> (2.6, 156.5) construction
  circle A7 centre (84.4, 160) radius 2.3
  line L22 (80.9, 163.5) -> (87.9, 163.5)
  line L23 (87.9, 163.5) -> (87.9, 156.5)
  line L24 (87.9, 156.5) -> (80.9, 156.5)
  line L25 (80.9, 156.5) -> (80.9, 163.5)
  line L26 (84.4, 163.5) -> (84.4, 156.5) construction
  line L27 (80.9, 160) -> (87.9, 160) construction
  circle A8 centre (84.4, 87.5) radius 2.3
  line L28 (80.9, 91) -> (87.9, 91)
  line L29 (87.9, 91) -> (87.9, 84)
  line L30 (87.9, 84) -> (80.9, 84)
  line L31 (80.9, 84) -> (80.9, 91)
  line L32 (84.4, 91) -> (84.4, 84) construction
  line L33 (80.9, 87.5) -> (87.9, 87.5) construction
  circle A9 centre (84.4, 15) radius 2.3
  line L34 (80.9, 18.5) -> (87.9, 18.5)
  line L35 (87.9, 18.5) -> (87.9, 11.5)
  line L36 (87.9, 11.5) -> (80.9, 11.5)
  line L37 (80.9, 11.5) -> (80.9, 18.5)
  line L38 (80.9, 15) -> (87.9, 15) construction
  line L39 (84.4, 18.5) -> (84.4, 11.5) construction
  line L40 (7.75, 148) -> (79.25, 148) construction
  line L41 (79.25, 148) -> (79.25, 0) construction
  line L42 (79.25, 0) -> (7.75, 0) construction
  line L43 (7.75, 0) -> (7.75, 148) construction
  line L44 (84.4, 160) -> (84.4, 87.5) construction
  line L45 (7.75, 6) -> (0, 6)
  line L46 (0, 6) -> (0, 10)
  line L47 (0, 10) -> (7.75, 10)
  line L48 (7.75, 10) -> (7.75, 6)
  line L49 (0, 172.5) -> (0, 2.5)
  line L50 (79.25, 6) -> (87, 6)
  line L51 (87, 6) -> (87, 10)
  line L52 (87, 10) -> (79.25, 10)
  line L53 (79.25, 10) -> (79.25, 6)
  line L54 (87, 2.5) -> (87, 172.5)
  line L55 (7.75, 137.5) -> (0, 137.5)
  line L56 (0, 137.5) -> (0, 142.5)
  line L57 (0, 142.5) -> (7.75, 142.5)
  line L58 (7.75, 142.5) -> (7.75, 137.5)
  line L59 (79.25, 137.5) -> (87, 137.5)
  line L60 (87, 137.5) -> (87, 142.5)
  line L61 (87, 142.5) -> (79.25, 142.5)
  line L62 (79.25, 142.5) -> (79.25, 137.5)
  line L63 (83.125, 137.5) -> (83.125, 142.5) construction
  line L64 (57, 148) -> (62, 148)
  line L65 (62, 148) -> (62, 175)
  line L66 (62, 175) -> (57, 175)
  line L67 (57, 175) -> (57, 148)
  line L68 (84.5, 175) -> (2.5, 175)
  line L69 (25, 148) -> (30, 148)
  line L70 (30, 148) -> (30, 175)
  line L71 (30, 175) -> (25, 175)
  line L72 (25, 175) -> (25, 148)
  circle A10 centre (2.6, 160) radius 1.75
  circle A11 centre (43.5, 165.5) radius 2
  circle A12 centre (43.5, 152.7) radius 2
  line L73 (12.75, 148) -> (22.75, 148)
  line L74 (22.75, 148) -> (22.75, 17)
  line L75 (22.75, 17) -> (12.75, 17)
  line L76 (12.75, 17) -> (12.75, 148)
  line L77 (64.25, 148) -> (74.25, 148)
  line L78 (74.25, 148) -> (74.25, 17)
  line L79 (74.25, 17) -> (64.25, 17)
  line L80 (64.25, 17) -> (64.25, 148)
  line L81 (12.75, 90) -> (22.75, 90)
  line L82 (22.75, 90) -> (22.75, 138)
  line L83 (22.75, 138) -> (12.75, 138)
  line L84 (12.75, 138) -> (12.75, 90)
  line L85 (22.75, 90) -> (12.5, 90)
  line L86 (12.5, 90) -> (12.5, 80)
  line L87 (12.5, 80) -> (22.75, 80)
  line L88 (22.75, 80) -> (22.75, 90)
  line L89 (22.75, 80) -> (12.5, 80)
  line L90 (12.5, 80) -> (12.5, 32)
  line L91 (12.5, 32) -> (22.75, 32)
  line L92 (22.75, 32) -> (22.75, 80)
  line L93 (22.75, 32) -> (12.5, 32)
  line L94 (12.5, 32) -> (12.5, 22)
  line L95 (12.5, 22) -> (22.75, 22)
  line L96 (22.75, 22) -> (22.75, 32)
  line L97 (64.25, 22) -> (74.5, 22)
  line L98 (74.5, 22) -> (74.5, 32)
  line L99 (74.5, 32) -> (64.25, 32)
  line L100 (64.25, 32) -> (64.25, 22)
  line L101 (74.25, 80) -> (64.5, 80)
  line L102 (64.5, 80) -> (64.5, 90)
  line L103 (64.5, 90) -> (74.25, 90)
  line L104 (74.25, 90) -> (74.25, 80)
  line L105 (64.25, 148) -> (74.5, 148)
  line L106 (74.5, 148) -> (74.5, 138)
  line L107 (74.5, 138) -> (64.25, 138)
  line L108 (64.25, 138) -> (64.25, 148)
  line L109 (72.5, 0) -> (84.5, 0)
  line L110 (2.5, 0) -> (14.5, 0)
  dimension "d234" = 4.6
  dimension "d235" = 7
  dimension "d236" = 7
  dimension "d250" = 4.6
  dimension "d251" = 7
  dimension "d252" = 7
  dimension "d253" = 4.6
  dimension "d254" = 7
  dimension "d255" = 7
  dimension "d256" = 4.6
  dimension "d257" = 7
  dimension "d258" = 7
  dimension "d259" = 4.6
  dimension "d260" = 7
  dimension "d261" = 7
  dimension "d262" = 4.6
  dimension "d263" = 7
  dimension "d264" = 7
  dimension "d268" = 71.5
  dimension "d269" = 148
  dimension "d270" = 2.4
  dimension "d283" = 4
  dimension "d285" = 4
  dimension "d288" = 5
  dimension "d289" = 5
  dimension "d290" = 5
  dimension "d291" = 25
  dimension "d292" = 5
  dimension "d293" = 25
  dimension "d299" = 3.5
  dimension "d322" = 4
  dimension "d323" = 4
  dimension "d324" = 11.9
  dimension "d325" = 12.8
  dimension "d328" = 10
  dimension "d329" = 131
  dimension "d330" = 5
  dimension "d331" = 10
  dimension "d332" = 131
  dimension "d333" = 5
  dimension "d334" = 10
  dimension "d336" = 10
  dimension "d338" = 10
  dimension "d339" = 5
  dimension "d340" = 48
  dimension "d341" = 10
  dimension "d342" = 5
  dimension "d343" = 10
  dimension "d344" = 48
  dimension "d345" = 10
  dimension "d396" = 6
  dimension "d397" = 6
  dimension "d447" = 7.75
  dimension "d448" = 14
  dimension "d449" = 14
  measures "d234" diameter of A4
  measures "d250" diameter of A5
  measures "d251" distance of origin
  measures "d253" diameter of A6
  measures "d254" distance of origin
  measures "d256" diameter of A7
  measures "d259" diameter of A8
  measures "d262" diameter of A9
  measures "d268" distance of origin
  measures "d270" distance of origin
  measures "d291" distance of L54 L65
  measures "d293" distance of L49 L72
  measures "d299" diameter of A10
  measures "d322" diameter of A11
  measures "d323" diameter of A12
  measures "d328" distance of origin
  measures "d330" distance of L43 L76
  measures "d332" distance of origin
  measures "d333" distance of L41 L78
  measures "d334" distance of L40 L83
  measures "d339" distance of L75 L95
  measures "d340" distance of L87 L91
  measures "d342" distance of L79 L97
  measures "d344" distance of L99 L101
  measures "d396" distance of L45 L110
  measures "d397" distance of L50 L109
  measures "d447" distance of L60 L62
  measures "d448" distance of L24 L61
  measures "d449" distance of L18 L57
extrude "Extrude19" add sketch "battery_screw" against normal blind 1.5 from surface at -2.4 contours A4 | L4 L6 L7 L49 | L4 L5 L6 L49 | A5 | L10 L12 L13 L49 | L10 L11 L12 L49 | A6 | L16 L18 L19 L49 | L16 L17 L18 L49 | A7 | L22 L24 L25 L54 | L22 L23 L24 L54 | A8 | L28 L30 L31 L54 | L28 L29 L30 L54 | A9 | L34 L36 L37 L54 | L34 L35 L36 L54 | A10 bodies 2
extrude "Extrude20" cut sketch "battery_screw" against normal blind 3.9 contours A4 | A5 | A6 | A7 | A8 | A9 | A10 bodies 2
chamfer "Chamfer3" distance 2 angle 45 6 edges at (0.4556, -23, 15.8317) (82.2556, -23, 15.8317) (82.2556, -23, 88.3317) (0.4556, -23, 88.3317) (0.4556, -23, 160.8317) (82.2556, -23, 160.8317) measured on face at (56.546, -23, 62.8405) measured on face at (56.546, -23, 62.8405) measured on face at (56.546, -23, 62.8405) measured on face at (56.546, -23, 62.8405) measured on face at (56.546, -23, 62.8405) measured on face at (56.546, -23, 62.8405) on bodies 2
fillet "Fillet9" radius 1 42 edges at (3.05, -20.6, 18.5) (6.1, -20.6, 15) (3.05, -20.6, 11.5) (0, -19.85, 11.5) (0, -19.85, 18.5) (3.05, -20.6, 84) (6.1, -20.6, 87.5) (3.05, -20.6, 91) (6.1, -19.85, 91) (6.1, -19.85, 84) (0, -19.85, 91) (0, -19.85, 84) (6.1, -19.85, 11.5) (6.1, -19.85, 18.5) (3.05, -20.6, 156.5) (6.1, -20.6, 160) (6.1, -19.85, 156.5) (0, -19.85, 156.5) (0, -19.85, 163.5) (3.05, -20.6, 163.5) (6.1, -19.85, 163.5) (87, -19.85, 156.5) (83.95, -20.6, 156.5) (80.9, -19.85, 156.5) (80.9, -20.6, 160) (80.9, -19.85, 163.5) (83.95, -20.6, 163.5) (87, -19.85, 163.5) (87, -19.85, 91) (83.95, -20.6, 91) (80.9, -19.85, 91) (80.9, -20.6, 87.5) (80.9, -19.85, 84) (83.95, -20.6, 84) (87, -19.85, 84) (87, -19.85, 18.5) (83.95, -20.6, 18.5) (80.9, -19.85, 18.5) (80.9, -20.6, 15) (80.9, -19.85, 11.5) (87, -19.85, 11.5) (83.95, -20.6, 11.5) on bodies 2
extrude "Extrude27" add sketch "headset_panel" against normal blind 2.4 contours L0 L16 L17 L18 L21 L24 L29 L30 | L16 L24 L26 L27 L29 | L0 L16 L18 L19 L23 L24 L30 L31 | L16 L21 L24 L29 L30 | L16 L23 L24 L30 L31 | L16 L24 L25 L26 L31 bodies 1
fillet "Fillet10" radius 2 4 edges at (24, 5.2, -1.2) (30, 5.2, -1.2) (30, -2, -1.2) (24, -2, -1.2) on bodies 1
extrude "Extrude22" add sketch "battery_screw" against normal blind 20 from surface at -2.4 contours L45 L46 L47 L48 L49 | L49 L55 L56 L57 L58 | L50 L51 L52 L53 L54 | L54 L59 L60 L61 L62 | L64 L65 L66 L67 L68 | L68 L69 L70 L71 L72 bodies 2
fillet "Fillet11" radius 1 22 edges at (79.25, -10.6, 6) (79.25, -10.6, 10) (87, -10.6, 10) (87, -10.6, 137.5) (79.25, -10.6, 137.5) (79.25, -10.6, 142.5) (87, -10.6, 142.5) (0, -10.6, 142.5) (7.75, -10.6, 142.5) (7.75, -10.6, 137.5) (0, -10.6, 137.5) (0, -10.6, 10) (7.75, -10.6, 10) (7.75, -10.6, 6) (62, -10.6, 148) (62, -10.6, 175) (30, -10.6, 175) (30, -10.6, 148) (57, -10.6, 148) (25, -10.6, 148) (57, -10.6, 175) (25, -10.6, 175) on bodies 2
extrude "Extrude24" cut sketch "battery_bottom" against normal up to surface (1.6 mm away) contours L0 L38 L39 L40 L41 bodies 3
fillet "Fillet12" radius 2 4 edges at (24, 1.2, 0.6) (24, 1.2, 8.1) (30, 1.2, 8.1) (30, 1.2, 0.6) on bodies 3
extrude "Extrude25" cut sketch "battery_screw" against normal up to surface (2.4 mm away) contours A11 | A12 bodies 2
extrude "Extrude26" add sketch "battery_screw" against normal blind 6.5 from surface at -2.4 contours L73 L74 L76 L83 | L74 L76 L81 L85 L87 L88 L89 | L74 L76 L91 L93 L95 L96 | L77 L78 L80 L105 L107 L108 | L78 L80 L97 L99 L100 | L78 L101 L102 L103 L104 bodies 2
fillet "Fillet13" radius 2.5 24 edges at (22.75, -17.35, 80) (12.75, -17.35, 80) (22.75, -17.35, 90) (12.75, -17.35, 90) (64.5, -17.35, 90) (74.25, -17.35, 90) (74.25, -17.35, 80) (64.25, -17.35, 32) (64.25, -17.35, 22) (12.75, -17.35, 22) (12.75, -17.35, 32) (22.75, -17.35, 32) (74.25, -17.35, 32) (64.25, -17.35, 138) (74.25, -17.35, 22) (22.75, -17.35, 22) (64.5, -17.35, 80) (22.75, -17.35, 138) (12.75, -17.35, 138) (74.25, -17.35, 138) (74.25, -17.35, 148) (64.25, -17.35, 148) (12.75, -17.35, 148) (22.75, -17.35, 148) on bodies 2
extrude "Extrude29" add sketch "electronics" along normal blind 2 from surface at 33 contours A12 A20 L47 L48 | L11 L27 L48 L50 L51 | L8 L24 L44 L45 L47 | A16 A20 L47 L48 | L15 L27 L48 L49 L50 | L12 L24 L45 L46 L47 | L11 L27 L64 L65 L66 | L8 L24 L36 L37 L39 | L15 L27 L64 L66 L67 | A13 A21 L39 L40 | L12 L24 L37 L38 L39 | L11 L27 L60 L62 L63 | L9 L25 L40 L42 L43 | A17 A21 L39 L40 | L15 L27 L60 L61 L62 | L13 L25 L40 L41 L42 | L11 L16 L18 L19 L27 | L9 L25 L56 L57 L58 | A15 L16 L23 A23 | L15 L16 L17 L18 L27 | L13 L25 L56 L58 L59 | L10 L20 L21 L23 L26 | A19 L16 L23 A23 | L9 L25 L52 L53 L54 | L14 L21 L22 L23 L26 | L13 L25 L52 L54 L55 | L10 L26 L28 L29 L31 | L9 L25 L32 L34 L35 | A14 A22 L31 L32 | L13 L25 L32 L33 L34 | A18 A22 L31 L32 bodies 1
extrude "Extrude30" add sketch "electronics" along normal blind 1.5 from surface at 35 contours A16 A20 L47 L48 | L15 L27 L48 L49 L50 | L12 L24 L45 L46 L47 | L15 L27 L64 L66 L67 | L12 L24 L37 L38 L39 | A17 A21 L39 L40 | L15 L27 L60 L61 L62 | L13 L25 L40 L41 L42 | L15 L16 L17 L18 L27 | L13 L25 L56 L58 L59 | A19 L16 L23 A23 | L14 L21 L22 L23 L26 | L13 L25 L52 L54 L55 | L13 L25 L32 L33 L34 | A18 A22 L31 L32 bodies 1
fillet "Fillet15" radius 1.5 23 edges at (0, 1, 170.5) (4.5, 1, 175) (4.5, 0.25, 173.5) (1.5, 0.25, 170.5) (85.5, 0.25, 170.5) (87, 1, 170.5) (87, 1, 4.5) (85.5, 0.25, 4.5) (82.5, 0.25, 1.5) (82.5, 1, 0) (4.5, 1, 0) (4.5, 0.25, 1.5) (0, 1, 4.5) (85.5, 0.25, 135) (85.5, 0.25, 130) (87, 1, 130) (87, 1, 135) (87, 1, 40) (87, 1, 45) (0, 1, 40) (0, 1, 45) (0, 1, 130) (0, 1, 135) on bodies 1
chamfer "Chamfer5" distance 1.5 angle 45 16 edges at (4.25, 2, 175) (0.7322, 2, 174.2678) (0, 2, 170.75) (87, 2, 170.75) (86.2678, 2, 174.2678) (83.5, 2, 175) (82.75, 2, 0) (86.2678, 2, 0.7322) (87, 2, 4.25) (0, 2, 4.25) (0.7322, 2, 0.7322) (4.25, 2, 0) (87, 2, 42.5) (87, 2, 132.5) (0, 2, 132.5) (0, 2, 42.5) on bodies 1
extrude "Extrude31" cut sketch "battery_bottom" against normal up to surface (1.6 mm away) contours A0 L0 L3 L43 | L3 L45 L46 L47 L48 | L0 A1 L1 L44 | L3 L49 L50 L51 L52 | L1 L53 L54 L55 L56 | L1 L57 L58 L59 L60 bodies 3
fillet "Fillet16" radius 2.5 20 edges at (0.6, 1.2, 6) (6, 1.2, 0.6) (86.4, 1.2, 6) (81, 1.2, 0.6) (0.6, 1.2, 46.1) (2.6, 1.2, 46.1) (2.6, 1.2, 39.1) (0.6, 1.2, 39.1) (0.6, 1.2, 136.1) (2.6, 1.2, 136.1) (2.6, 1.2, 129.1) (0.6, 1.2, 129.1) (86.4, 1.2, 39.1) (84.4, 1.2, 39.1) (84.4, 1.2, 46.1) (86.4, 1.2, 46.1) (84.4, 1.2, 136.1) (86.4, 1.2, 136.1) (86.4, 1.2, 129.1) (84.4, 1.2, 129.1) on bodies 3
fillet "Fillet17" radius 5 2 edges at (10, -2, -1.2) (77, -2, -1.2) on bodies 1
extrude "Extrude33" cut sketch "headset_panel" against normal blind 2.4 contours L0 L16 L17 L18 L21 L24 L29 L30 | L16 L24 L26 L27 L29 | L0 L16 L18 L19 L23 L24 L30 L31 | L16 L21 L24 L29 L30 | L16 L22 L24 L26 L28 L29 L31 | L16 L23 L24 L30 L31 | L16 L24 L25 L26 L31 bodies 2
extrude "Extrude35" cut sketch "battery_conn_hole" against normal blind 2.4 contours L0 L29 L30 L32 L35 | L30 L31 L32 L33 L35 L36 | L13 L18 L30 L33 L35 | L13 L18 L33 L34 L35 | L0 L21 L22 L24 L27 | L22 L23 L24 L25 L27 L28 | L15 L20 L22 L25 L27 | L15 L20 L25 L26 L27 bodies 1
extrude "Extrude38" add sketch "oled_panel" against normal blind 2 from surface at -5 separate body contours L4 L66 L67 L80 | L4 L14 L47 L66 L67 L80 | L4 L5 L8 L41 L59 L60 L66 L77 L79 L80 | L4 L14 L47 L66 L77 L80 | L11 L13 L14 L15 A2 L47 L66 L67 A7 L80 | L2 L21 L45 L74 L79 | L2 L6 L7 L49 L50 L74 L77 L79 | L5 L8 L41 L77 | L5 L6 L7 L41 L77 L79 | L59 L60 L79 | L13 L14 L47 L66 L80 | L11 L67 L68 | L2 L21 L45 L74 L78 | L2 L71 L74 L77 L78 | L18 L45 L74 L79 | L13 L47 L66 L77 L80 | L13 L15 L65 L66 L80 | L11 L12 L13 L15 A2 L65 L68 A7 | L2 L21 L45 L71 L78 | L2 L71 L78 | L18 L21 L45 L74 L78 | L18 L21 L45 L74 | L18 L74 L78 | L18 L73 L78 | L13 L15 L65 | L18 L19 L20 L21 L45 L71 L72 L78 L82 | L49 L50 L77 | L18 L19 L73 L82 | L12 L65 L68 | L19 L72 L73 | L20 L71 L72 makes body 4
fillet "Fillet19" radius 4 4 edges at (63.7686, 2.7504, 171.4) (67.7338, 9.4635, 171.4) (19.2644, 29.4032, 171.4) (23.2032, 36.1356, 171.4) on bodies 4
extrude "Extrude39" add sketch "oled_panel" against normal blind 1 from surface at -2.4 contours L30 L31 L32 L33 | A10 bodies 1
extrude "Extrude6" cut sketch "oled_panel" against normal blind 1 from surface at -2.4 contours L30 L31 L32 L33 bodies 1
chamfer "Chamfer6" distance 1 angle 45 1 edges at (4.2767, 13.8838, 175) on bodies 1
chamfer "Chamfer7" distance 1 angle 45 8 edges at (23.703, 35, 149.5848) (72.703, 35, 149.5848) (72.703, 35, 91.5848) (23.703, 35, 91.5848) (23.203, 35, 62.0848) (48.203, 35, 47.0848) (45.203, 35, 27.0848) (22.203, 35, 27.0848) on bodies 1
named bodies: "main_body", "battery_case", "battery_bottom", "oled_holder"
